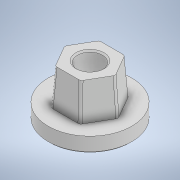
# Autodesk Inventor part: TeflonHolderWasher
Saved by Autodesk Inventor 2020 (Build 240168000, 168)
## iProperties
Created: 2020-01-16
Part Number: TeflonHolderWasher
Material: Generic
Document SubType Name: Modeling
Designer: Parker
Density: 1 g/cm^3
Appearance: Default
Author: Parker
Autodesk Inventor part; units mm, degrees
ref_plane "YZ Plane" through (0, 0, 0) normal (1, 0, 0) x (0, 1, 0)
ref_plane "XZ Plane" through (0, 0, 0) normal (0, 1, 0) x (-1, 0, 0)
ref_plane "XY Plane" through (0, 0, 0) normal (0, 0, 1) x (1, 0, 0)
sketch "Sketch1" plane through (0, 0, 0) normal (0, 1, 0) x (-1, 0, 0)
  circle A0 centre (0, 0) radius 7
  circle A1 centre (0, 0) radius 2.1
  dimension "d0" = 14
  dimension "d1" = 4.2
  constraints: 2 centre point, 2 coincident
  measures "d0" diameter of A0
  measures "d1" diameter of A1
extrude "Extrusion1" add sketch "Sketch1" along normal blind 2.5
sketch "Sketch2" plane through (0, 2.5, 0) normal (0, 1, 0) x (1, 0, 0)
  circle A0 centre (0, 0) radius 2.1
  line L0 (4.7343, 0) -> (2.3671, -4.1)
  line L1 (2.3671, -4.1) -> (-2.3671, -4.1)
  line L2 (-2.3671, -4.1) -> (-4.7343, 0)
  line L3 (-4.7343, 0) -> (-2.3671, 4.1)
  line L4 (-2.3671, 4.1) -> (2.3671, 4.1)
  line L5 (2.3671, 4.1) -> (4.7343, 0)
  dimension "d10" = 2
  dimension "d11" = 4.2
  constraints: 12 end point, 1 centre point, 1 coincident, 13 other
  measures "d10" distance edge to line of A0 L4
  measures "d11" diameter of A0
extrude "Extrusion2" add sketch "Sketch2" along normal blind 6
chamfer "Chamfer1" distance 0.25 angle 45 3 edges at (7, 0, 0) (-2.1, 8.5, 0) (2.1, 0, 0)
draft "FaceDraft1" angle 4 pull direction (0, 1, 0) faces at (3.1562, 4.5, 2.7333) (-0.789, 4.5, 4.1) (3.9452, 4.5, -1.3667) (-3.9452, 4.5, 1.3667) (-3.1562, 4.5, -2.7333) (0.789, 4.5, -4.1) fixed edges at (3.5507, 2.5, 2.05) (0, 2.5, 4.1) (3.5507, 2.5, -2.05) (-3.5507, 2.5, 2.05) (-3.5507, 2.5, -2.05) (0, 2.5, -4.1)
fillet "Fillet1" radius 0.5 6 edges at (-2.246, 5.5, 3.8902) (2.246, 5.5, 3.8902) (4.492, 5.5, 0) (2.246, 5.5, -3.8902) (-2.246, 5.5, -3.8902) (-4.492, 5.5, 0)
body "Solid1"
